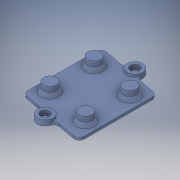
# Autodesk Inventor part: Membrane - Boutons
Saved by Autodesk Inventor 2019 (Build 230136000, 136)
## iProperties
Created: 2019-04-18
Part Number: Membrane - Boutons
Material: Caoutchouc
Document SubType Name: Modeling
Designer: Sébastien DI MERCURIO
Density: 0.93 g/cm^3
Appearance: Caoutchouc - Bleu
Author: Sébastien DI MERCURIO
Autodesk Inventor part; units mm, degrees
ref_plane "YZ Plane" through (0, 0, 0) normal (1, 0, 0) x (0, 1, 0)
ref_plane "XZ Plane" through (0, 0, 0) normal (0, 1, 0) x (-1, 0, 0)
ref_plane "XY Plane" through (0, 0, 0) normal (0, 0, 1) x (1, 0, 0)
sketch "Esquisse2" plane through (0, 0, 0) normal (0, 1, 0) x (-1, 0, 0)
  line L0 (13, 12.5) -> (13, -17.5)
  line L1 (13, -17.5) -> (-13, -12.5)
  line L2 (-13, -12.5) -> (-13, 17.5)
  line L3 (-13, 17.5) -> (13, 12.5)
  point P0 (0, 0)
  dimension "d0" = 30
  dimension "d1" = 26
  dimension "d2" = 13
  dimension "d4" = 5
  dimension "d5" = 30
  dimension "d11" = 12.5
  constraints: 8 end point, 1 parallel, 1 vertical
  measures "d0" distance of L0.start L0.end
  measures "d1" distance between parallel lines of L2 L0
  measures "d2" distance from line of point (0, 0) L0
  measures "d4" vertical distance of L1.end L0.end
  measures "d5" distance of L1.end L2.end
  measures "d11" vertical distance of point (0, 0) L0.start
extrude "Extrusion1" add sketch "Esquisse2" along normal blind 1
sketch "Esquisse3" plane through (0, 1, 0) normal (0, 1, 0) x (1, 0, 0)
  circle A0 centre (-1, -16.2192) radius 1.75
  circle A1 centre (1, 16.2192) radius 1.75
  line L0 (-1, -16.2192) -> (0, 0) construction
  line L1 (0, 0) -> (1, 16.2192) construction
  line L2 (13, -17.5) -> (13, 12.5) construction
  circle A2 centre (-1, -16.2192) radius 3
  circle A3 centre (1, 16.2192) radius 3
  dimension "d8" = 3.5
  dimension "d9" = 3.5
  dimension "d10" = 36
  dimension "d13" = 12
  dimension "d14" = 6
  dimension "d15" = 6
  constraints: 4 centre point, 4 end point, 2 coincident, 2 collinear
  measures "d8" diameter of A0
  measures "d9" diameter of A1
  measures "d13" distance from line of L2 L1.end
  measures "d14" diameter of A2
  measures "d15" diameter of A3
extrude "Extrusion2" add sketch "Esquisse3" along normal blind 1 and the other way blind 1
fillet "Congé1" radius 2 4 edges at (-3.3509, 0.5, 14.3556) (1.8745, 0.5, 15.3605) (-1.8745, 0.5, -15.3605) (3.3509, 0.5, -14.3556)
fillet "Congé2" radius 2 4 edges at (13, 0.5, -12.5) (13, 0.5, 17.5) (-13, 0.5, 12.5) (-13, 0.5, -17.5)
sketch "Esquisse4" plane through (0, 1, 0) normal (0, 1, 0) x (1, 0, 0)
  circle A0 centre (-8.3657, -6.9951) radius 3.5
  circle A1 centre (-8.3657, 10.0049) radius 3.5
  circle A2 centre (8.3657, 6.9951) radius 3.5
  circle A3 centre (8.3657, -10.0049) radius 3.5
  line L0 (0, -25) -> (0, 25) construction
  line L1 (-13.9609, 0) -> (15.5775, 0) construction
  line L2 (-13, 15.0787) -> (-13, -10.848) construction
  circle A4 centre (-1, -16.2192) radius 1.75 construction
  line L3 (-8.3657, -6.9951) -> (0, -6.9951) construction
  line L4 (8.3657, -10.0049) -> (0, -10.0049) construction
  line L5 (-8.3657, 10.0049) -> (0, 10.0049) construction
  line L6 (8.3657, 6.9951) -> (0, 6.9951) construction
  line L7 (-7.4081, -6.9951) -> (-7.4081, 0) construction
  line L8 (8.3657, 6.9951) -> (8.3657, 0) construction
  point P0 (0, 0)
  dimension "d22" = 7
  dimension "d23" = 7
  dimension "d24" = 7
  dimension "d25" = 7
  dimension "d26" = 17
  dimension "d27" = 17
  dimension "d28" = 24
  dimension "d29" = 24
  dimension "d30" = 13
  dimension "d32" = 50
  dimension "d33" = 25
  dimension "d34" = 25
  constraints: 16 end point, 7 point on line, 5 perpendicular, 4 centre point, 3 parallel, 2 horizontal, 1 vertical
  measures "d22" diameter of A0
  measures "d23" diameter of A1
  measures "d24" diameter of A2
  measures "d25" diameter of A3
  measures "d26" distance of L5.start L3.start
  measures "d27" distance of L6.start L4.start
  measures "d30" distance between parallel lines of L0 L2
  measures "d32" distance of L0.end L0.start
  measures "d33" distance of point (0, 0) L0.start
  measures "d34" distance from line of L0.start L1
extrude "Extrusion3" add sketch "Esquisse4" along normal blind 1.5
sketch "Esquisse5" plane through (-8.3657, 2.5, 6.9951) normal (0, 1, 0) x (1, 0, 0)
  circle A0 centre (0, 0) radius 2.5
  circle A1 centre (0, 17) radius 2.5
  circle A2 centre (16.7314, -3.0099) radius 2.5
  circle A3 centre (16.7314, 13.9901) radius 2.5
  circle A4 centre (16.7314, 13.9901) radius 3.5 projected
  circle A5 centre (0, 17) radius 3.5 projected
  circle A6 centre (16.7314, -3.0099) radius 3.5 projected
  circle A7 centre (0, 0) radius 3.5 projected
  point P0 (8.3657, 6.9951)
  dimension "d37" = 5
  dimension "d38" = 5
  dimension "d39" = 5
  dimension "d40" = 5
  constraints: 4 centre point, 4 concentric
  measures "d37" diameter of A0
  measures "d38" diameter of A1
  measures "d39" diameter of A2
  measures "d40" diameter of A3
extrude "Extrusion4" add sketch "Esquisse5" along normal blind 2 contours A0 | A1 | A2 | A3
chamfer "Chanfrein1" distance 1 distance2 1.5 1 edges at (-11.8657, 2.5, 6.9951) measured on face at (-5.2329, 2.5, 7.2743)
chamfer "Chanfrein2" distance 1 distance2 1.5 1 edges at (-11.8657, 2.5, -10.0049) measured on face at (-5.2329, 2.5, -9.7257)
chamfer "Chanfrein3" distance 1 distance2 1.5 1 edges at (4.8657, 2.5, 10.0049) measured on face at (11.4743, 2.5, 10.4836)
chamfer "Chanfrein4" distance 1 distance2 1.5 1 edges at (4.8657, 2.5, -6.9951) measured on face at (11.4985, 2.5, -6.7159)
equation "\"d2\" = 0.5 * d1"
equation "\"d5\" = d0"
equation "\"d11\" = 0.5 * d0 - 0.5 * d4"
equation "\"d9\" = d8"
equation "\"d15\" = d14"
equation "\"d23\" = d22"
equation "\"d24\" = d22"
equation "\"d25\" = d22"
equation "\"d27\" = d26"
equation "\"d28\" = d26 + d22"
equation "\"d29\" = d28"
equation "\"d33\" = 0.5 * d32"
equation "\"d34\" = d33"
equation "\"d38\" = d37"
equation "\"d39\" = d37"
equation "\"d40\" = d37"
